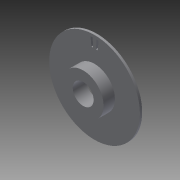
# Autodesk Inventor part: SmallPositionDisk
Saved by Autodesk Inventor 2015 (Build 190159000, 159)
## iProperties
Created: 2017-01-31
Part Number: SmallPositionDisk
Material: Generic
Document SubType Name: Modeling
Designer: Ernest
Density: 1 g/cm^3
Appearance: Default
Author: Ernest
Autodesk Inventor part; units mm, degrees
ref_plane "YZ Plane" through (0, 0, 0) normal (1, 0, 0) x (0, 1, 0)
ref_plane "XZ Plane" through (0, 0, 0) normal (0, 1, 0) x (-1, 0, 0)
ref_plane "XY Plane" through (0, 0, 0) normal (0, 0, 1) x (1, 0, 0)
sketch "Sketch1" plane through (0, 0, 0) normal (0, 1, 0) x (-1, 0, 0)
  circle A0 centre (0, 0) radius 20
  line L0 (0, 0) -> (20, 0)
  circle A1 centre (0, 0) radius 4.6
  dimension "d1" = 40
  dimension "d6" = 9.2
  constraints: 2 end point, 1 centre point, 1 horizontal, 1 horizontal alignment, 2 other
  measures "d6" diameter of A1
extrude "Extrusion1" add sketch "Sketch1" along normal blind 6
sketch "Sketch2" plane through (0, 0, 0) normal (0, -1, 0) x (1, 0, 0)
  circle A0 centre (0, 0) radius 4.6 projected
  circle A1 centre (0, 0) radius 20 projected
  circle A2 centre (0, 0) radius 9
  circle A3 centre (0, 0) radius 20
  dimension "d7" = 18
  constraints: 2 centre point, 2 coincident
  measures "d7" diameter of A2
extrude "Extrusion2" cut sketch "Sketch2" against normal blind 5 contours A1
sketch "Sketch3" plane through (0, 6, 0) normal (0, 1, 0) x (1, 0, 0)
  circle A0 centre (0, 0) radius 4.6 projected
  circle A1 centre (0, 0) radius 20 projected
  line L0 (0, 0) -> (0, -20)
  circle A2 centre (0, 0) radius 20 projected
  line L1 (2.4, -13.5) -> (2.4, -20)
  line L2 (2.4, -20) -> (-2.4, -20)
  line L3 (-2.4, -20) -> (-2.4, -13.5)
  line L4 (-2.4, -13.5) -> (2.4, -13.5)
  line L5 (2.4, -13.5) -> (-2.4, -20) construction
  line L6 (2.4, -20) -> (-2.4, -13.5) construction
  line L7 (0.25, -18.6) -> (1.75, -18.6)
  line L8 (1.75, -18.6) -> (1.75, -14.9)
  line L9 (1.75, -14.9) -> (0.25, -14.9)
  line L10 (0.25, -14.9) -> (0.25, -18.6)
  line L11 (-0.25, -18.6) -> (-1.75, -18.6)
  line L12 (-1.75, -18.6) -> (-1.75, -14.9)
  line L13 (-1.75, -14.9) -> (-0.25, -14.9)
  line L14 (-0.25, -14.9) -> (-0.25, -18.6)
  arc A3 (-0.8149, -18.6644) -> (-1.75, -18.6) centre (0, 0) ccw
  arc A4 (-0.65, -14.8879) -> (-1.3959, -14.8366) centre (0, 0) ccw
  line L15 (0, 0) -> (-0.65, -14.8879)
  line L16 (0, 0) -> (0.65, -14.8879)
  line L17 (0, 0) -> (-1.3959, -14.8366)
  line L18 (0, 0) -> (1.3959, -14.8366)
  arc A5 (-1.3959, -14.8366) -> (-0.65, -14.8879) centre (0, 0) ccw
  arc A6 (-1.3886, -18.6305) -> (-0.8149, -18.6644) centre (0, 0) ccw
  arc A7 (-1.75, -18.6) -> (-1.3886, -18.6305) centre (0, 0) ccw
  line L19 (-0.65, -14.8879) -> (-0.8149, -18.6644)
  line L20 (-1.3959, -14.8366) -> (-1.75, -18.6)
  line L21 (1.3959, -14.8366) -> (1.75, -18.6)
  line L22 (0.65, -14.8879) -> (0.8149, -18.6644)
  point P0 (0, -16.75)
  dimension "d10" = 0
  dimension "d11" = 4.8
  dimension "d12" = 6.5
  dimension "d13" = 1.5
  dimension "d14" = 3.7
  dimension "d17" = 1.4
  dimension "d40" = 2
  dimension "d41" = 0.25
  dimension "d76" = 5
  dimension "d77" = 2.5
  constraints: 46 end point, 19 point on circle, 7 parallel, 6 point on line, 5 centre point, 3 perpendicular, 2 coincident, 2 horizontal, 2 midpoint, 2 vertical alignment, 1 collinear, 1 vertical, 2 other
  measures "d10" distance from line of L2 L0.end
  measures "d11" distance of L1.end L2.end
  measures "d12" distance of L2.end L3.end
  measures "d13" distance of L7.start L7.end
  measures "d14" distance of L7.end L8.end
  measures "d17" distance between parallel lines of L11 L2
  measures "d40" distance between parallel lines of L14 L8
  measures "d41" distance between parallel lines of L0 L10
  measures "d76" angle of L15 L16
  measures "d77" angle of L0 L16
extrude "Extrusion4" cut sketch "Sketch3" against normal blind 10 contours A5 L19 L13 L20 | L21 L9 L22 A4 | L13 L19 L11 L20 | L21 L7 L22 L9 | L11 L19 A6 A7 | A3 L22 L7
equation "\"d17\" = -0.5 * d14 + 0.5 * d12"
equation "\"d41\" = -0.5 * d13 + 0.5 * d40"
equation "\"d77\" = 0.5 * d76"
body "Solid1"
